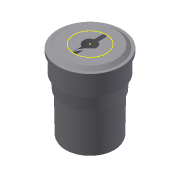
# Autodesk Inventor part: Practice Trash Can by Jessica
Saved by Autodesk Inventor 2015 (Build 190159000, 159)
## iProperties
Created: 2015-01-04
Part Number: Practice Trash Can by Jessica
Material: Generic
Document SubType Name: Modeling
Designer: Peter
Density: 1 g/cm^3
Appearance: Default
Author: Peter
Autodesk Inventor part; units mm, degrees
ref_plane "YZ Plane" through (0, 0, 0) normal (1, 0, 0) x (0, 1, 0)
ref_plane "XZ Plane" through (0, 0, 0) normal (0, 1, 0) x (-1, 0, 0)
ref_plane "XY Plane" through (0, 0, 0) normal (0, 0, 1) x (1, 0, 0)
sketch "Sketch1" plane through (0, 0, 0) normal (0, 0, 1) x (1, 0, 0)
  line L0 (0, 0) -> (222.25, 0)
  line L1 (222.25, 0) -> (222.25, 12.7)
  line L2 (222.25, 12.7) -> (225.425, 12.7)
  line L3 (228.6, 15.875) -> (228.6, 28.575)
  arc A0 (225.425, 12.7) -> (228.6, 15.875) centre (225.425, 15.875) ccw
  line L4 (228.6, 28.575) -> (234.1467, 373.3979)
  line L5 (234.1467, 373.3979) -> (246.8467, 373.3979)
  line L6 (246.8467, 373.3979) -> (255.134, 500.3979)
  line L7 (255.134, 500.3979) -> (274.184, 500.3979)
  line L8 (274.184, 500.3979) -> (274.184, 664.6429)
  line L9 (274.184, 664.6429) -> (293.234, 664.6429)
  line L10 (293.234, 664.6429) -> (293.234, 699.5679)
  line L11 (293.234, 699.5679) -> (267.834, 699.5679)
  line L12 (267.834, 699.5679) -> (236.084, 724.9679)
  line L13 (236.084, 724.9679) -> (153.534, 724.9679)
  line L14 (153.534, 724.9679) -> (148.7715, 728.7779)
  line L15 (148.7715, 728.7779) -> (0, 728.7779)
  line L16 (0, 728.7779) -> (0, 0) construction
  line L17 (0, 728.7779) -> (0, 0) construction
  line L18 (0, 728.7779) -> (0, 0)
  point P0 (228.6, 12.7)
  dimension "d0" = 222.25
  dimension "d1" = 12.7
  dimension "d2" = 6.35
  dimension "d3" = 15.875
  dimension "d4" = 3.175
  dimension "d5" = 12.7
  dimension "d6" = 127
  dimension "d7" = 19.05
  dimension "d9" = 19.05
  dimension "d10" = 34.925
  dimension "d11" = 25.4
  dimension "d12" = 25.4
  dimension "d13" = 31.75
  dimension "d14" = 82.55
  dimension "d15" = 4.7625
  dimension "d16" = 728.7778
  constraints: 38 end point, 6 horizontal, 4 vertical, 3 parallel, 2 perpendicular, 2 point on circle, 2 point on line, 2 tangent, 1 centre point, 1 collinear
  measures "d0" distance of L0.start L0.end
  measures "d1" distance of L0.end L1.end
  measures "d2" distance of L1.end point (228.6, 12.7)
  measures "d3" distance of point (228.6, 12.7) L3.end
  measures "d4" radius of A0
  measures "d5" distance of L4.end L5.end
  measures "d6" vertical distance of L5.end L6.end
  measures "d7" distance of L6.end L7.end
  measures "d9" distance of L8.end L9.end
  measures "d10" distance of L9.end L10.end
  measures "d11" distance of L10.end L11.end
  measures "d12" vertical distance of L12.end L11.end
  measures "d13" horizontal distance of L11.end L12.end
  measures "d14" distance of L12.end L13.end
  measures "d15" horizontal distance of L14.end L13.end
  measures "d16" distance of L0.start L15.end
revolve "Revolution1" add sketch "Sketch1" angle 360 about axis through (0, 728.7779, 0) along (0, -1, 0)
shell "Shell1" thickness 5.08 removed faces 1 at (-54.4916, 0, -94.5607)
fillet "Fillet1" radius 3.175 1 edges at (-293.234, 699.5679, 0)
sketch "Sketch3" plane through (0, 728.7779, 0) normal (0, 1, 0) x (1, 0, 0)
  circle A0 centre (0, 0) radius 148.7715 projected
sketch "Sketch4" plane through (0, 728.7779, 0) normal (0, 1, 0) x (1, 0, 0)
  circle A0 centre (0, 0) radius 148.7715 projected
sketch "Sketch5" plane through (0, 728.7779, 0) normal (0, 1, 0) x (1, 0, 0)
  circle A0 centre (0, 0) radius 148.7715 projected
sketch "Sketch6" plane through (0, 728.7779, 0) normal (0, 1, 0) x (1, 0, 0)
  circle A0 centre (0, 0) radius 148.7715 projected
  circle A1 centre (0, 0) radius 60.325
  line L0 (0, -125.4125) -> (0, 125.4125) construction
  line L1 (-19.05, -125.4125) -> (-19.05, 125.4125)
  line L2 (19.05, 125.4125) -> (19.05, -125.4125)
  arc A2 (-19.05, -125.4125) -> (19.05, -125.4125) centre (0, -125.4125) ccw
  arc A3 (19.05, 125.4125) -> (-19.05, 125.4125) centre (0, 125.4125) ccw
  dimension "d20" = 120.65
  dimension "d21" = 38.1
  dimension "d22" = 250.825
  constraints: 8 end point, 4 point on circle, 4 tangent, 3 centre point, 1 coincident, 1 midpoint, 1 parallel, 1 vertical
  measures "d20" diameter of A1
  measures "d21" distance between parallel lines of L2 L1
  measures "d22" distance of L0.start L0.end
extrude "Extrusion1" cut sketch "Sketch6" against normal through all contours A1 L2 | L2 A1 L1 | A1 L1 A3 L2 | L2 A2 L1 A1 | L1 A1
body "Solid1"
